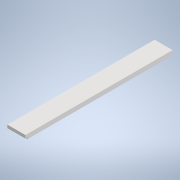
# Autodesk Inventor part: Arcade_MonitorStand
Saved by Autodesk Inventor 2022 (Build 260153000, 153)
## iProperties
Created: 2023-12-22
Part Number: Arcade_MonitorStand
Material: Generic
Document SubType Name: Modeling
Designer: Petr Černý
Density: 1 g/cm^3
Appearance: Default
Author: Petr Černý
Autodesk Inventor part; units mm, degrees
ref_plane "YZ Plane" through (0, 0, 0) normal (1, 0, 0) x (0, 1, 0)
ref_plane "XZ Plane" through (0, 0, 0) normal (0, 1, 0) x (-1, 0, 0)
ref_plane "XY Plane" through (0, 0, 0) normal (0, 0, 1) x (1, 0, 0)
sketch "Sketch1" plane through (0, 0, 0) normal (0, 1, 0) x (-1, 0, 0)
  line L0 (28.8538, 64.9138) -> (-31.1462, 64.9138)
  line L1 (-31.1462, 64.9138) -> (-31.1462, -425.0862)
  line L2 (-31.1462, -425.0862) -> (28.8538, -425.0862)
  line L3 (28.8538, -425.0862) -> (28.8538, 64.9138)
  point P0 (0, 0)
  dimension "d0" = 60
  dimension "d1" = 490
  constraints: 8 end point, 2 parallel, 1 horizontal, 1 perpendicular
  measures "d0" distance of L2.end L1.end
  measures "d1" distance of L1.end L0.end
extrude "Extrusion1" add sketch "Sketch1" along normal blind 15
sketch "Sketch2" plane through (-28.8538, 0, 64.9138) normal (0, 0, 1) x (1, 0, 0)
  line L0 (60, 0) -> (0, 0) projected
  line L1 (0, 0) -> (60, 0)
  line L2 (60, 0) -> (60, 5)
  line L3 (60, 5) -> (0, 5)
  line L4 (0, 5) -> (0, 0)
  point P0 (28.8538, 0)
  point P1 (60, 0)
  dimension "d4" = 60
  dimension "d5" = 5
  constraints: 8 end point, 2 parallel, 1 horizontal, 1 perpendicular
  measures "d4" distance of L3.end L2.end
  measures "d5" distance of L2.end L1.end
extrude "Extrusion2" cut sketch "Sketch2" against normal blind 7
sketch "Sketch3" plane through (31.1462, 0, -425.0862) normal (0, 0, -1) x (-1, 0, 0)
  line L0 (0, 0) -> (60, 0) projected
  line L1 (0, 0) -> (60, 0)
  line L2 (60, 0) -> (60, 5)
  line L3 (60, 5) -> (0, 5)
  line L4 (0, 5) -> (0, 0)
  point P0 (31.1462, 0)
  point P1 (60, 0)
  dimension "d8" = 60
  dimension "d9" = 5
  constraints: 8 end point, 2 parallel, 1 horizontal, 1 perpendicular
  measures "d8" distance of L3.end L2.end
  measures "d9" distance of L2.end L1.end
extrude "Extrusion3" cut sketch "Sketch3" against normal blind 7
body "Solid1"
